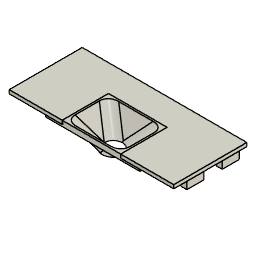
smartie_hopper (Autodesk Fusion 360 archive; units mm, degrees)
design "Smartie Hopper" references "Colour Detection Mechanism Top Panel Placeholder", "Smartie Hopper", "Colour Detection Mechanism Top Panel", "Back Label"
part number: 2026-04-09-18-25-13-653
Autodesk Fusion 360 part; units mm, degrees
sketch "Bottom opening" plane through (0, 0, 0) normal (0, 0, 1) x (1, 0, 0)
  line L0 (0, 0) -> (30, 0)
  line L1 (30, 0) -> (30, 30)
  line L2 (30, 30) -> (0, 30)
  line L3 (0, 30) -> (0, 0)
  line L4 (-4, 34) -> (34, 34)
  line L5 (34, 34) -> (34, -4)
  line L6 (34, -4) -> (-4, -4)
  line L7 (-4, -4) -> (-4, 34)
  dimension "d3" = 30
  dimension "d4" = 30
  dimension "d5" = 4
  dimension "d6" = 4
  dimension "d7" = 4
  dimension "d8" = 4
  constraint horizontal L0
  constraint vertical L1
  constraint horizontal L2
  constraint vertical L3
  constraint coincident L0.start L3.end
  constraint horizontal L4
  constraint vertical L5
  constraint horizontal L6
  constraint vertical L7
  measures "d3" distance of L0.start L0.end
  measures "d4" distance of L0.end L1.end
  measures "d5" distance of L2 L4
  measures "d6" distance of L0 L6
  measures "d7" distance of L1 L5
  measures "d8" distance of L3 L7
ref_plane "WorkPlane1" through (0, 0, 34) normal (0, 0, 1) x (1, 0, 0)
sketch "Top opening" plane through (0, 0, 34) normal (0, 0, 1) x (1, 0, 0)
  line L0 (30, 30) -> (0, 30)
  line L1 (30, 0) -> (30, 30)
  line L2 (0, 0) -> (30, 0)
  line L3 (0, 30) -> (0, 0)
  line L4 (-4, 34) -> (34, 34)
  line L5 (34, -4) -> (-4, -4)
  line L6 (34, 34) -> (34, -4)
  line L7 (-4, -4) -> (-4, 34)
  line L8 (-29.5, 51.5) -> (60.5, 51.5)
  line L9 (60.5, 51.5) -> (60.5, -18.5)
  line L10 (60.5, -18.5) -> (-29.5, -18.5)
  line L11 (-29.5, -18.5) -> (-29.5, 51.5)
  line L12 (-32.5, 54.5) -> (63.5, 54.5)
  line L13 (63.5, 54.5) -> (63.5, -21.5)
  line L14 (63.5, -21.5) -> (-32.5, -21.5)
  line L15 (-32.5, -21.5) -> (-32.5, 54.5)
  line L16 (-33.5, 55.5) -> (64.5, 55.5)
  line L17 (64.5, 55.5) -> (64.5, -22.5)
  line L18 (64.5, -22.5) -> (-33.5, -22.5)
  line L19 (-33.5, -22.5) -> (-33.5, 55.5)
  dimension "d14" = 3
  dimension "d15" = 4
  dimension "d16" = 3
  dimension "d17" = 4
  dimension "d18" = 90
  dimension "d19" = 70
  dimension "d20" = 3
  dimension "d21" = 4
  dimension "d22" = 3
  dimension "d23" = 4
  dimension "d24" = 25.5
  dimension "d25" = 26.5
  dimension "d26" = 17.5
  dimension "d27" = 14.5
  constraint horizontal L8
  constraint vertical L9
  constraint horizontal L10
  constraint vertical L11
  constraint horizontal L12
  constraint vertical L13
  constraint horizontal L14
  constraint vertical L15
  constraint horizontal L16
  constraint vertical L17
  constraint horizontal L18
  constraint vertical L19
  measures "d14" distance of L9 L13
  measures "d15" distance of L9 L17
  measures "d16" distance of L11 L15
  measures "d17" distance of L11 L19
  measures "d18" distance of L8.start L8.end
  measures "d19" distance of L8.end L9.end
  measures "d20" distance of L8 L12
  measures "d21" distance of L8 L16
  measures "d22" distance of L10 L14
  measures "d23" distance of L10 L18
  measures "d24" distance of L7 L11
  measures "d25" distance of L6 L9
  measures "d26" distance of L4 L8
  measures "d27" distance of L5 L10
loft "Loft1" add profiles "Top opening", "Bottom opening" section 1 contours L8 L9 L10 L11 | L12 L13 L14 L15 | L16 L17 L18 L19 section 2 contours L0 L1 L2 L3 | L4 L5 L6 L7
extrude "Extrude1" cut sketch "Top opening" against normal blind 6 contours L16 L17 L18 L19
extrude "Extrude4" add 1 faces at (-0.5, 3.8333, 34) along direction (0, 0, -1) blind 6
sketch "Support lip" plane through (63.5, 0, 0) normal (1, 0, 0) x (0, 1, 0)
  line L0 (54.5, 28) -> (54.5, 34)
  line L1 (54.5, 34) -> (-21.5, 34)
  line L2 (-21.5, 34) -> (-21.5, 28)
  line L3 (-21.5, 28) -> (84.5, 28)
  line L4 (84.5, 28) -> (84.5, 23)
  line L5 (84.5, 23) -> (-21.5, 23)
  line L6 (-21.5, 23) -> (-21.5, 28)
  line L7 (-21.5, 28) -> (54.5, 28)
  line L8 (-21.5, 28) -> (16.5, 28)
  line L9 (16.5, 28) -> (16.5, 23)
  line L10 (16.5, 23) -> (-21.5, 23)
  line L11 (-21.5, 23) -> (-21.5, 28)
  dimension "d31" = 6
  dimension "d34" = 5
  dimension "d35" = 30
  dimension "d50" = 38
  constraint horizontal L3
  constraint vertical L4
  constraint horizontal L5
  constraint vertical L6
  constraint collinear L2 L6
  constraint horizontal L8
  constraint vertical L9
  constraint horizontal L10
  constraint vertical L11
  constraint coincident L5 L9.end
  constraint coincident L2.end L3.start
  measures "d31" distance of L1 L3
  measures "d34" distance of L2.end L5.end
  measures "d35" horizontal distance of L0.end L3.end
  measures "d50" distance of L9 L11
extrude "Extrude2" add sketch "Support lip" along normal blind 30 and the other way blind 126 contours L3 L5 L6 L7 L8 L9 L10 L11
extrude "Extrude5" add sketch "Support lip" against normal blind 78 from surface at -48 contours L3 L4 L5 L7 L9
fillet "Fillet4" radius 5 5 edges at (93.5, 16.5, 25.5) (93.5, -21.5, 25.5) (15.5, 84.5, 25.5) (-62.5, 84.5, 25.5) (-62.5, -21.5, 25.5)
loft "Loft2" cut profiles "Top opening", "Bottom opening" section 1 contours L8 L9 L10 L11 section 2 contours L0 L1 L2 L3
fillet "Fillet3" radius 19.5 4 edges at (-14.75, 40.75, 17) (-14.75, -9.25, 17) (45.25, -9.25, 17) (45.25, 40.75, 17)
fillet "Fillet5" radius 24.5 4 edges at (-13.9779, -10.2574, 11.5) (-13.9779, 41.2721, 11.5) (46.5588, 42.8529, 14) (44.3162, -10.2574, 11.5)
sketch "3D printing angle" plane through (93.5, 0, 0) normal (1, 0, 0) x (0, 1, 0)
  line L0 (-16.5, 28) -> (-16.5, 23)
  line L1 (-16.5, 23) -> (11.5, 23)
  line L2 (11.5, 23) -> (11.5, 28)
  line L3 (11.5, 28) -> (-16.5, 28)
  line L4 (54.5, 28) -> (54.5, 34)
  line L5 (54.5, 34) -> (-21.5, 34)
  line L6 (-21.5, 34) -> (-21.5, 28)
  line L7 (-21.5, 28) -> (16.5, 28)
  line L8 (16.5, 28) -> (54.5, 28)
  line L9 (-16.5, 23) -> (-21.5, 23)
  line L10 (-16.5, 23) -> (-16.5, 28)
  line L11 (-21.5, 28) -> (-16.5, 28)
  line L12 (-21.5, 28) -> (-21.5, 23)
  line L13 (11.5, 28) -> (16.5, 28)
  line L14 (11.5, 28) -> (11.5, 23)
  line L15 (16.5, 23) -> (11.5, 23)
  line L16 (16.5, 23) -> (16.5, 28)
  line L17 (-21.5, 34) -> (-19.5604, 23)
  dimension "d58" = 10
  constraint coincident L5.end L6.start
  constraint coincident L9 L17.end
  measures "d58" angle of L6 L17
extrude "Extrude6" cut sketch "3D printing angle" against normal blind 156 contours L7 L9 L11 L12 L17 | L6 L7 L11 L17
equation "bottom_outlet_size = 30 mm" comment "The side lengths of the bottom opening of the Smartie Hopper."
equation "hopper_wall_thickness = 4 mm" comment "The thickness of the hopper walls used for the \"loft\" function."
equation "d3 = bottom_outlet_size"
equation "d4 = bottom_outlet_size"
equation "d5 = hopper_wall_thickness"
equation "d6 = hopper_wall_thickness"
equation "d7 = hopper_wall_thickness"
equation "d8 = hopper_wall_thickness"
equation "hopper_height = 34 mm" comment "Distance between the top and bottom openings of the Smartie Hopper."
equation "d10 = hopper_height"
equation "acrylic_thickness = 3 mm" comment "Thickness of the clear acrylic panels used for the Unsorted Smarties Holder."
equation "top_outlet_width = 90 mm" comment "The width of the top opening of the Smartie Hopper."
equation "top_outlet_depth = 70 mm" comment "The depth of the top opening of the Smartie Hopper."
equation "d14 = acrylic_thickness"
equation "d15 = hopper_wall_thickness"
equation "d16 = acrylic_thickness"
equation "d17 = hopper_wall_thickness"
equation "d18 = top_outlet_width"
equation "d19 = top_outlet_depth"
equation "d20 = acrylic_thickness"
equation "d21 = hopper_wall_thickness"
equation "d22 = acrylic_thickness"
equation "d23 = hopper_wall_thickness"
equation "d24 = ( top_outlet_width - ( bottom_outlet_size + 2 * hopper_wall_thickness ) ) / 2 - outlet_alignment_offset_width"
equation "d26 = ( top_outlet_depth - ( bottom_outlet_size + 2 * hopper_wall_thickness ) ) / 2 + outlet_alignment_offset_depth"
equation "MDF_thickness = 6 mm" comment "Thickness of the MDF panels used for the construction of the mini arcade game enclosure."
equation "d29 = -MDF_thickness"
equation "d31 = MDF_thickness"
equation "support_lip_width = 30 mm" comment "The depth that the suport lip should extend beneath the Colour Detection Mechanism Top Panel."
equation "support_lip_thickness = 5 mm" comment "The thickness of the support lip."
equation "d34 = support_lip_thickness"
equation "d35 = support_lip_width"
equation "d36 = support_lip_width"
equation "d38 = ( top_outlet_width + 2 * acrylic_thickness ) + support_lip_width"
equation "d46 = -MDF_thickness"
equation "d50 = ( top_outlet_depth / 2 ) + acrylic_thickness"
equation "d51 = -( top_outlet_width / 2 ) - acrylic_thickness"
equation "d52 = -( top_outlet_width / 2 ) - acrylic_thickness - support_lip_width"
equation "d59 = -( top_outlet_width + 2 * acrylic_thickness + 2 * support_lip_width )"
equation "outlet_alignment_offset_depth = 1.5 mm" comment "A parameter for ensuring that the bottom outlet of the Smartie Hopper is directly above the hole of the Smartie Arm depth-wise."
equation "outlet_alignment_offset_width = 0.5 mm" comment "A parameter for ensuring that the bottom outlet of the Smartie Hopper is directly above the hole of the Smartie Arm width-wise."

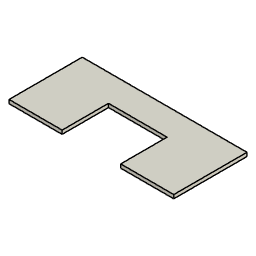
design "Colour Detection Mechanism Top Panel"
part number: 2025-05-13-09-48-31-121
Autodesk Fusion 360 part; units mm, degrees
sketch "Sorting Mechanism Top Panel" plane through (0, 0, 0) normal (0, 0, 1) x (1, 0, 0)
  line L0 (0, 0) -> (270, 0)
  line L1 (270, 0) -> (270, 120)
  line L2 (270, 120) -> (0, 120)
  line L3 (0, 120) -> (0, 0)
  dimension "d1" = 270
  dimension "d2" = 120
  constraint horizontal L0
  constraint vertical L1
  constraint horizontal L2
  constraint vertical L3
  constraint coincident L0.start L3.end
  measures "d1" distance of L0.start L0.end
  measures "d2" distance of L0.end L1.end
extrude "Extrude1" add sketch "Sorting Mechanism Top Panel" along normal blind 6
sketch "Smartie Hopper Hole" plane through (0, 0, 6) normal (0, 0, 1) x (-1, 0, 0)
  line L0 (0, -120) -> (0, 0)
  line L1 (0, 0) -> (-270, 0)
  line L2 (-270, 0) -> (-270, -120)
  line L3 (-270, -120) -> (0, -120)
  line L4 (-87, -76) -> (-183, -76)
  line L5 (-183, -76) -> (-183, 0)
  line L6 (-183, 0) -> (-87, 0)
  line L7 (-87, 0) -> (-87, -76)
  dimension "d7" = 96
  dimension "d9" = 76
  dimension "d10" = 87
  dimension "d11" = 87
  constraint horizontal L4
  constraint vertical L5
  constraint horizontal L6
  constraint vertical L7
  constraint collinear L1 L6
  measures "d7" distance of L4.start L4.end
  measures "d9" distance of L4.end L5.end
  measures "d10" distance of L0 L7
  measures "d11" distance of L2 L5
extrude "Extrude2" cut sketch "Smartie Hopper Hole" against normal blind 6 contours L1 L4 L5 L6 L7
equation "d3 = MDF_thickness"
equation "acrylic_thickness = 3 mm" comment "Thickness of the clear acrylic panels"
equation "MDF_thickness = 6 mm" comment "Thickness of the MDF panels"
equation "d7 = smarties_hopper_width + 2 * acrylic_thickness"
equation "smarties_hopper_width = 90 mm" comment "Width of the Smarties hopper"
equation "d9 = smarties_hopper_depth + 2 * acrylic_thickness"
equation "d10 = ( 270 mm - ( smarties_hopper_width + 2 * acrylic_thickness ) ) / 2"
equation "d14 = -MDF_thickness"
equation "smarties_hopper_depth = 70 mm" comment "Depth of the Smarties hopper"
named bodies: "Sorting Mechanism Top Panel"

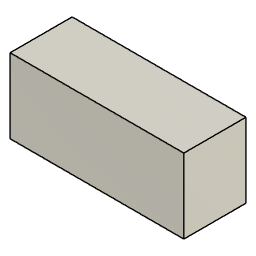
design "Colour Detection Mechanism Top Panel Placeholder"
part number: 2025-05-14-09-44-42-407
Autodesk Fusion 360 part; units mm, degrees
sketch "Sorting Mechanism Top Panel Placeholder" plane through (0, 0, 0) normal (0, 0, 1) x (1, 0, 0)
  line L0 (0, 0) -> (28, 0)
  line L1 (28, 0) -> (28, 10)
  line L2 (28, 10) -> (0, 10)
  line L3 (0, 10) -> (0, 0)
  dimension "d1" = 10
  dimension "d2" = 28
  constraint horizontal L0
  constraint vertical L1
  constraint horizontal L2
  constraint vertical L3
  constraint coincident L0.start L3.end
  measures "d1" distance of L0.end L1.end
  measures "d2" distance of L0.start L0.end
extrude "Extrude1" add sketch "Sorting Mechanism Top Panel Placeholder" along normal blind 12
named bodies: "Sorting Mechanism Top Panel Placeholder"

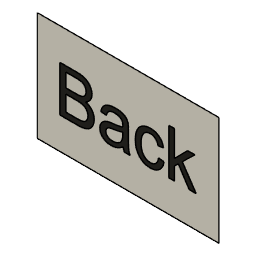
design "Back Label"
part number: 2025-04-13-10-14-33-970
Autodesk Fusion 360 part; units mm, degrees
sketch "Sticker" plane through (0, 0, 0) normal (0, 1, 0) x (1, 0, 0)
  line L0 (0, 0) -> (20, 0)
  line L1 (20, 0) -> (20, -12)
  line L2 (20, -12) -> (0, -12)
  line L3 (0, -12) -> (0, 0)
  dimension "d1" = 12
  dimension "d2" = 20
  constraint horizontal L0
  constraint vertical L1
  constraint horizontal L2
  constraint vertical L3
  constraint coincident L0.start L3.end
  measures "d1" distance of L0.end L1.end
  measures "d2" distance of L0.start L0.end
extrude "Extrude1" add sketch "Sticker" along normal blind 0.01 makes body 1
sketch "Text" plane through (0, 0, 0) normal (0, -1, 0) x (1, 0, 0)
  line L0 (20, 12) -> (0, 12)
  line L1 (0, 12) -> (0, 0)
  line L2 (0, 0) -> (20, 0)
  line L3 (20, 0) -> (20, 12)
  line L4 (0, 0) -> (20, 0) construction
  line L5 (20, 0) -> (20, 12) construction
  line L6 (20, 12) -> (0, 12) construction
  line L7 (0, 12) -> (0, 0) construction
  dimension "d5" = 5
  text T0 "Back" font "Arial" height 5 align centre middle in box 20 x 12 at (0, 0) x (1, 0) y (0, 1) spacing 1 kerned
  constraint coincident L2.end
  constraint coincident L0.end
extrude "Extrude2" add sketch "Text" along normal blind 0.01 separate body text T0 makes body 2 at (14.6982, 0, 5.8829) makes body 3 at (11.2962, 0, 4.2151) makes body 4 at (9.8356, 0, 4.5282) makes body 5 at (2.7257, 0, 5.9363)
equation "d8 = 'Back'"
named bodies: "Sticker", "Text 4", "Text 3", "Text 2", "Text 1"
